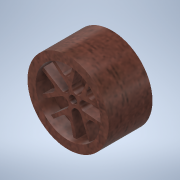
# Autodesk Inventor part: 前輪 改
Saved by Autodesk Inventor 2020.2 (Build 242310000, 310)
## iProperties
Created: 2020-03-19
Part Number: 前輪 改
Material: 一般
Document SubType Name: Modeling
Designer: 黃柏維
Density: 1 g/cm^3
Appearance: 預設
Author: 黃柏維
Autodesk Inventor part; units mm, degrees
ref_plane "YZ Plane" through (0, 0, 0) normal (1, 0, 0) x (0, 1, 0)
ref_plane "XZ Plane" through (0, 0, 0) normal (0, 1, 0) x (-1, 0, 0)
ref_plane "XY Plane" through (0, 0, 0) normal (0, 0, 1) x (1, 0, 0)
sketch "草圖1" plane through (0, 0, 0) normal (0, 0, 1) x (1, 0, 0)
  circle A0 centre (0, 0) radius 25
  circle A1 centre (0, 0) radius 2.1
  dimension "d0" = 50
  dimension "d1" = 4.2
  constraints: 2 centre point, 2 coincident
  measures "d0" diameter of A0
  measures "d1" diameter of A1
extrude "擠出1" add sketch "草圖1" along normal blind 27
sketch "Sketch2" plane through (0, 0, 27) normal (0, 0, 1) x (1, 0, 0)
  circle A0 centre (0, 0) radius 25 projected
  circle A1 centre (0, 0) radius 20
  dimension "d4" = 40
  constraints: 1 centre point, 1 coincident
  measures "d4" diameter of A1
extrude "Extrusion2" cut sketch "Sketch2" against normal blind 3 contours A1
sketch "Sketch4" plane through (0, 0, 24) normal (0, 0, 1) x (1, 0, 0)
  circle A0 centre (0, 0) radius 2.1
  constraints: 1 centre point, 1 coincident
extrude "Extrusion3" add sketch "Sketch4" against normal up to surface (24 mm away)
sketch "Sketch5" plane through (0, 0, 24) normal (0, 0, 1) x (1, 0, 0)
  arc A0 (6.7648, 2.9908) -> (6.7648, -2.9908) centre (7, 0) ccw
  circle A1 centre (0, 0) radius 20 projected
  line L0 (19.5959, 4) -> (6.7648, 2.9908)
  line L1 (19.5959, -4) -> (6.7648, -2.9908)
  line L2 (9.8597, 17.4008) -> (4.9348, 5.5095)
  arc A2 (-0.754, 7.3579) -> (4.9348, 5.5095) centre (2.1631, 6.6574) ccw
  line L3 (2.2512, 19.8729) -> (-0.754, 7.3579)
  line L4 (-13.5023, 14.7543) -> (-3.7149, 6.3958)
  arc A3 (-7.2307, 1.5566) -> (-3.7149, 6.3958) centre (-5.6631, 4.1145) ccw
  line L5 (-18.2046, 8.2821) -> (-7.2307, 1.5566)
  line L6 (-18.2046, -8.2821) -> (-7.2307, -1.5566)
  arc A4 (-3.7149, -6.3958) -> (-7.2307, -1.5566) centre (-5.6631, -4.1145) ccw
  line L7 (-13.5023, -14.7543) -> (-3.7149, -6.3958)
  line L8 (2.2512, -19.8729) -> (-0.754, -7.3579)
  arc A5 (4.9348, -5.5095) -> (-0.754, -7.3579) centre (2.1631, -6.6574) ccw
  line L9 (9.8597, -17.4008) -> (4.9348, -5.5095)
  line L10 (11.7075, 16.6355) -> (8.7645, 9.5294)
  line L11 (19.4391, 5.9938) -> (11.7714, 5.3907)
  line L12 (19.0893, -5.9663) -> (19.4391, -5.9938)
  arc A6 (8.7645, 9.5294) -> (11.7714, 5.3907) centre (11.5361, 8.3815) ccw
  circle A7 centre (0, 0) radius 20 projected
  line L13 (0.3065, 20.3399) -> (-1.4893, 12.8611)
  arc A8 (-6.3547, 11.2802) -> (-1.4893, 12.8611) centre (-4.4064, 13.5616) ccw
  line L14 (-12.2035, 16.2751) -> (-6.3547, 11.2802)
  line L15 (-19.2496, 6.5769) -> (-12.6918, 2.5578)
  arc A9 (-12.6918, -2.5578) -> (-12.6918, 2.5578) centre (-14.2595, 0) ccw
  line L16 (-19.2496, -6.5769) -> (-12.6918, -2.5578)
  line L17 (-12.2035, -16.2751) -> (-6.3547, -11.2802)
  arc A10 (-1.4893, -12.8611) -> (-6.3547, -11.2802) centre (-4.4064, -13.5616) ccw
  line L18 (0.3065, -20.3399) -> (-1.4893, -12.8611)
  line L19 (11.7075, -16.6355) -> (8.7645, -9.5294)
  arc A11 (11.7714, -5.3907) -> (8.7645, -9.5294) centre (11.5361, -8.3815) ccw
  line L20 (19.4391, -5.9938) -> (11.7714, -5.3907)
  point P0 (19.0893, 5.9663)
  point P1 (11.5732, 16.3113)
  point P2 (11.5732, -16.3113)
  point P3 (-11.9367, -16.0473)
  point P4 (0.2246, -19.9987)
  point P5 (-18.9505, 6.3936)
  point P6 (-18.9505, -6.3936)
  point P7 (0.2246, 19.9987)
  point P8 (-11.9367, 16.0473)
  dimension "d9" = 6
  dimension "d12" = 360
  dimension "d14" = 2
  dimension "d15" = 2
  dimension "d16" = 3
  dimension "d19" = 360
  constraints: 42 end point, 23 point on circle, 10 centre point, 4 tangent, 83 other
  measures "d9" diameter of A0
  measures "d14" distance between parallel lines of L2 L10
  measures "d15" distance between parallel lines of L0 L11
  measures "d16" radius of A6
extrude "Extrusion4" cut sketch "Sketch5" against normal blind 6 contours L0 A1 L1 A0 | L11 A6 L10 A1 | A1 L19 A11 L20 | L2 A2 L3 A1 | A1 L8 A5 L9 | L13 A8 L14 A1 | A1 L17 A10 L18 | L4 A3 L5 A1 | A1 L6 A4 L7 | L15 A9 L16 A1
sketch "Sketch9" plane through (0, 0, 0) normal (0, 0, -1) x (-1, 0, 0)
  circle A0 centre (0, 0) radius 2.1
  dimension "d38" = 4.2
  constraints: 1 centre point, 1 coincident
  measures "d38" diameter of A0
extrude "Extrusion7" cut sketch "Sketch9" against normal blind 18
sketch "Sketch10" plane through (0, 0, 24) normal (0, 0, 1) x (1, 0, 0)
  circle A0 centre (0, 0) radius 2.1 projected
  circle A1 centre (0, 0) radius 2.5
  dimension "d41" = 5
  constraints: 1 centre point, 1 coincident
  measures "d41" diameter of A1
extrude "Extrusion8" cut sketch "Sketch10" against normal blind 3 contours A0 | A1
